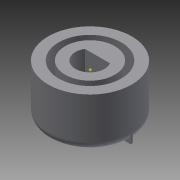
# Autodesk Inventor part: knob
Saved by Autodesk Inventor 2014 (Build 180170000, 170)
## iProperties
Created: 2013-09-15
Part Number: knob
Material: Generic
Document SubType Name: Modeling
Designer: stephen
Density: 1 g/cm^3
Appearance: Default
Author: stephen
Autodesk Inventor part; units mm, degrees
ref_plane "YZ Plane" through (0, 0, 0) normal (1, 0, 0) x (0, 1, 0)
ref_plane "XZ Plane" through (0, 0, 0) normal (0, 1, 0) x (-1, 0, 0)
ref_plane "XY Plane" through (0, 0, 0) normal (0, 0, 1) x (1, 0, 0)
sketch "Sketch1" plane through (0, 0, 0) normal (0, 0, 1) x (1, 0, 0)
  circle A0 centre (2.5244, 2.0294) radius 10
  point P0 (0, 0)
  dimension "d0" = 20
  constraints: 1 centre point
  measures "d0" diameter of A0
extrude "Extrusion1" add sketch "Sketch1" along normal blind 3
sketch "Sketch2" plane through (2.5244, 2.0294, 3) normal (0, 0, 1) x (1, 0, 0)
  circle A0 centre (0, 0) radius 10 projected
  circle A1 centre (0, 0) radius 7.5
  point P0 (-2.5244, -2.0294)
  dimension "d3" = 15
  constraints: 1 centre point, 1 coincident
  measures "d3" diameter of A1
extrude "Extrusion2" add sketch "Sketch2" along normal blind 6.9
sketch "Sketch3" plane through (2.5244, 2.0294, 3) normal (0, 0, 1) x (1, 0, 0)
  circle A0 centre (0, 0) radius 7.5 projected
  circle A1 centre (0, 0) radius 5.95
  arc A2 (-3.0017, 1.8) -> (3.0017, 1.8) centre (0, 0) ccw
  line L0 (0, 1.8) -> (3.0017, 1.8)
  line L1 (0, 1.8) -> (-3.0017, 1.8)
  line L2 (0, 1.8) -> (0, -3.5)
  point P0 (-2.5244, -2.0294)
  dimension "d6" = 11.9
  dimension "d7" = 7
  dimension "d18" = 5.3
  constraints: 6 end point, 3 point on circle, 2 centre point, 2 coincident, 1 collinear
  measures "d6" diameter of A1
  measures "d7" diameter of A2
  measures "d18" distance of L0.start L2.end
extrude "Extrusion3" add sketch "Sketch3" along normal blind 6.9 contours A1
fillet "Fillet1" radius 2 1 edges at (-7.4756, 2.0294, 0)
sketch "Sketch4" plane through (2.5244, 2.0294, 0) normal (0, 0, -1) x (-1, 0, 0)
  circle A0 centre (0, 0) radius 8 projected
  line L0 (-8, 0) -> (-7.9961, 0.25)
  line L1 (-7.9961, 0.25) -> (-7.9961, -0.25)
  line L2 (-7.9961, -0.25) -> (-9.9703, -0.25)
  line L3 (-9.9703, -0.25) -> (-9.9703, 0.25)
  line L4 (-9.9703, 0.25) -> (-7.9961, 0.25)
  point P0 (2.5244, -2.0294)
  dimension "d12" = 0.25
  dimension "d13" = 0.5
  constraints: 10 end point, 3 point on circle, 2 parallel, 1 perpendicular
  measures "d12" distance of L0.start L0.end
  measures "d13" distance of L0.end L1.end
extrude "Extrusion4" add sketch "Sketch4" against normal blind 1.85 contours A0 L2 L3 L4
sketch "Sketch5" plane through (0, 0, 0) normal (0, 0, -1) x (-1, 0, 0)
  line L0 (-10.5205, 2.2794) -> (-12.4947, 2.2794) projected
  line L1 (-12.4947, 2.2794) -> (-10.5205, 2.2794)
  line L2 (-10.5205, 2.2794) -> (-10.5205, 1.7794)
  line L3 (-10.5205, 1.7794) -> (-12.4947, 1.7794)
  line L4 (-12.4947, 1.7794) -> (-12.4947, 2.2794)
  point P0 (0, 0)
  constraints: 8 end point, 3 equal length, 1 perpendicular
extrude "Extrusion5" add sketch "Sketch5" along normal blind 0.35
sketch "Sketch7" plane through (2.5244, 2.0294, 9.9) normal (0, 0, 1) x (1, 0, 0)
  arc A0 (-3.0017, 1.8) -> (3.0017, 1.8) centre (0, 0) ccw projected
  line L0 (-3.0017, 1.8) -> (3.0017, 1.8) projected
  circle A1 centre (0, 0) radius 5.95 projected
  line L1 (3.0017, 1.8) -> (3.0017, 3.9445)
  point P0 (-2.5244, -2.0294)
  constraints: 2 end point, 1 perpendicular
extrude "Extrusion6" add sketch "Sketch7" along normal blind 2
sketch "Sketch8" plane through (2.5244, 2.0294, 9.9) normal (0, 0, 1) x (1, 0, 0)
  circle A0 centre (0, 0) radius 7.5 projected
  circle A1 centre (0, 0) radius 10 projected
  circle A2 centre (0, 0) radius 7.5
  circle A3 centre (0, 0) radius 10
  point P0 (-2.5244, -2.0294)
  constraints: 2 centre point, 2 coincident, 2 concentric
extrude "Extrusion7" add sketch "Sketch8" along normal blind 2
body "Solid1"
